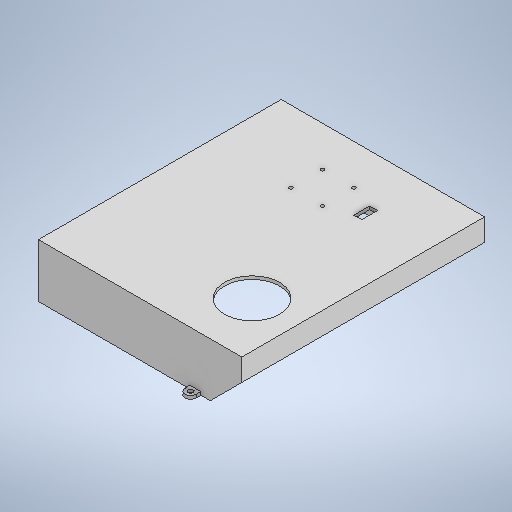
# Autodesk Inventor part: Część3
Saved by Autodesk Inventor 2025.2 (Build 292293000, 293)
## iProperties
Created: 2026-03-22
Part Number: Część3
Material: Ogólny
Document SubType Name: Modeling
Designer: janla
Density: 1 g/cm^3
Appearance: Domyślna
Author: janla
Autodesk Inventor part; units mm, degrees
ref_plane "YZ Plane" through (0, 0, 0) normal (1, 0, 0) x (0, 1, 0)
ref_plane "XZ Plane" through (0, 0, 0) normal (0, 1, 0) x (-1, 0, 0)
ref_plane "XY Plane" through (0, 0, 0) normal (0, 0, 1) x (1, 0, 0)
sketch "Szkic1" plane through (0, 0, 0) normal (0, 1, 0) x (-1, 0, 0)
  line L0 (-55.4115, -11.4249) -> (69.5885, -11.4249)
  line L1 (69.5885, -11.4249) -> (69.5885, -161.4249)
  line L2 (69.5885, -161.4249) -> (-55.4115, -161.4249)
  line L3 (-55.4115, -161.4249) -> (-55.4115, -11.4249)
  line L4 (-57.4115, -9.4249) -> (71.5885, -9.4249)
  line L5 (71.5885, -9.4249) -> (71.5885, -163.4249)
  line L6 (71.5885, -163.4249) -> (-57.4115, -163.4249)
  line L7 (-57.4115, -163.4249) -> (-57.4115, -9.4249)
  line L8 (-55.4115, -86.4249) -> (-60.9115, -86.4249)
  circle A0 centre (-60.9115, -86.4249) radius 1.65
  circle A1 centre (-60.9115, -86.4249) radius 3.5
  line L9 (-60.9115, -82.9249) -> (-57.4115, -82.9249)
  line L10 (-60.9115, -89.9249) -> (-57.4115, -89.9249)
  line L11 (-60.9115, -86.4249) -> (-27.9115, -86.4249)
  line L12 (-27.9115, -86.4249) -> (-27.9115, -166.4249)
  line L13 (-27.9115, -166.4249) -> (-27.9115, -6.4249)
  circle A2 centre (-27.9115, -6.4249) radius 1.65
  circle A3 centre (-27.9115, -166.4249) radius 1.65
  circle A4 centre (-27.9115, -6.4249) radius 3.5
  circle A5 centre (-27.9115, -166.4249) radius 3.5
  line L14 (-24.4115, -166.4249) -> (-24.4115, -163.4249)
  line L15 (-31.4115, -166.4249) -> (-31.4115, -163.4249)
  line L16 (-24.4115, -6.4249) -> (-24.4115, -9.4249)
  line L17 (-31.4115, -6.4249) -> (-31.4115, -9.4249)
  line L18 (7.0885, -9.4249) -> (7.0885, -161.4249)
  line L19 (69.5885, -11.4249) -> (42.5885, -11.4249)
  point P0 (0, 0)
  dimension "d0" = 125
  dimension "d1" = 150
  dimension "d2" = 2
  dimension "d3" = 2
  dimension "d4" = 2
  dimension "d5" = 2
  dimension "d6" = 5.5
  dimension "d7" = 3.3
  dimension "d8" = 33
  dimension "d9" = 80
  dimension "d10" = 160
  dimension "d11" = 3.3
  dimension "d12" = 3.3
  dimension "d13" = 7
  dimension "d14" = 7
  dimension "d33" = 27
  constraints: 40 end point, 12 point on line, 7 perpendicular, 6 centre point, 6 coincident, 6 point on circle, 4 horizontal, 4 parallel, 3 midpoint, 1 tangent
  measures "d0" distance between parallel lines of L1 L3
  measures "d1" distance between parallel lines of L0 L2
  measures "d2" distance between parallel lines of L5 L1
  measures "d3" distance between parallel lines of L0 L4
  measures "d4" distance between parallel lines of L6 L2
  measures "d5" distance between parallel lines of L3 L7
  measures "d6" distance of L8.start L8.end
  measures "d7" diameter of A0
  measures "d8" distance of L11.start L11.end
  measures "d9" distance of L11.end L12.end
  measures "d10" distance of L12.end L13.end
  measures "d11" diameter of A2
  measures "d12" diameter of A3
  measures "d13" diameter of A4
  measures "d14" diameter of A5
  measures "d33" distance of L0.end L19.end
extrude "Wyciągnięcie proste1" add sketch "Szkic1" along normal blind 2 contours L0 L18 L4 L5 L6 A5 L12 L2 L1 | L0 L13 A4 L4 L18 | L0 L3 L8 L7 L4 A4 L13 | A4 L4 L13 | L13 L4 A4 | L4 A4 L16 | L12 A5 L6 L7 L8 L3 L2 | L4 A4 | L4 L17 A4 | A5 L6 L12 | L12 L6 A5 | A1 L9 L7 | A1 | L7 L10 A1 | L14 A5 L6 | L6 A5 | A5 L15 L6
sketch "Szkic2" plane through (0, 2, 0) normal (0, 1, 0) x (1, 0, 0)
  line L0 (57.4115, 9.4249) -> (57.4115, 82.9249) projected
  line L1 (24.4115, 163.4249) -> (-71.5885, 163.4249) projected
  line L2 (57.4115, 9.4249) -> (-71.5885, 9.4249)
  line L3 (-71.5885, 9.4249) -> (-71.5885, 163.4249)
  line L4 (-71.5885, 163.4249) -> (57.4115, 163.4249)
  line L5 (57.4115, 163.4249) -> (57.4115, 9.4249)
  line L6 (55.4115, 11.4249) -> (-69.5885, 11.4249) projected
  line L7 (-69.5885, 11.4249) -> (55.4115, 11.4249)
  line L8 (55.4115, 11.4249) -> (55.4115, 161.4249)
  line L9 (55.4115, 161.4249) -> (-69.5885, 161.4249)
  line L10 (-69.5885, 161.4249) -> (-69.5885, 11.4249)
  point P0 (0, 0)
  point P1 (55.4115, 11.4249)
  constraints: 16 end point, 4 parallel, 2 horizontal, 2 perpendicular
extrude "Wyciągnięcie proste2" add sketch "Szkic2" along normal blind 30
sketch "Szkic3" plane through (0, 32, 0) normal (0, 1, 0) x (1, 0, 0)
  line L0 (57.4115, 9.4249) -> (57.4115, 163.4249) projected
  line L1 (-71.5885, 163.4249) -> (-71.5885, 9.4249) projected
  line L2 (57.4115, 163.4249) -> (-71.5885, 163.4249)
  line L3 (-71.5885, 163.4249) -> (-71.5885, 9.4249)
  line L4 (-71.5885, 9.4249) -> (57.4115, 9.4249)
  line L5 (57.4115, 9.4249) -> (57.4115, 163.4249)
  point P0 (0, 0)
  point P1 (-71.5885, 163.4249)
  point P2 (57.4115, 9.4249)
  constraints: 8 end point, 2 parallel, 1 horizontal, 1 perpendicular
extrude "Wyciągnięcie proste3" add sketch "Szkic3" along normal blind 2
sketch "Szkic5" plane through (57.4115, 0, -89.9249) normal (1, 0, 0) x (0, 0, -1)
  line L0 (0, 0) -> (-7, 0) projected
  line L1 (-7, 0) -> (0, 0)
  line L2 (0, 0) -> (0, 14)
  line L3 (0, 14) -> (-7, 14)
  line L4 (-7, 14) -> (-7, 0)
  line L5 (-80.5, 0) -> (-80.5, 2) projected
  line L6 (-80.5, 2) -> (-78.5, 2)
  line L7 (-78.5, 0) -> (-78.5, 32) projected
  line L8 (-7, 14) -> (-78.5, 14)
  line L9 (-78.5, 14) -> (-78.5, 2)
  line L10 (-78.5, 2) -> (-7, 2)
  line L11 (-7, 2) -> (-7, 14)
  line L12 (73.5, 0) -> (73.5, 34) projected
  line L13 (73.5, 2) -> (71.5, 2)
  line L14 (71.5, 0) -> (71.5, 32) projected
  line L15 (0, 14) -> (71.5, 14)
  line L16 (71.5, 14) -> (71.5, 2)
  line L17 (71.5, 2) -> (0, 2)
  line L18 (0, 2) -> (0, 14)
  line L19 (-7, 2) -> (-78.5, 2)
  line L20 (-78.5, 2) -> (-78.5, 0)
  line L21 (-78.5, 0) -> (-7, 0)
  line L22 (-7, 0) -> (-7, 2)
  line L23 (0, 2) -> (71.5, 2)
  line L24 (71.5, 2) -> (71.5, 0)
  line L25 (71.5, 0) -> (0, 0)
  line L26 (0, 0) -> (0, 2)
  point P0 (-89.9249, 0)
  point P1 (71.5, 14)
  point P2 (-78.5, 14)
  dimension "d24" = 14
  constraints: 44 end point, 10 parallel, 7 horizontal, 5 perpendicular, 3 point on line
  measures "d24" distance between parallel lines of L0 L3
extrude "Wyciągnięcie proste5" cut sketch "Szkic5" along normal mid plane 20
chamfer "Faza1" distance 20 angle 45 1 edges at (57.4115, 0, -10.4249)
sketch "Szkic6" plane through (-71.5885, 0, -163.4249) normal (-1, 0, 0) x (0, 0, 1)
  line L0 (0, 0) -> (154, 0) projected
  line L1 (154, 34) -> (0, 34) projected
  line L2 (0, 0) -> (154, 34)
  line L3 (0, 0) -> (0, 34) projected
  line L4 (154, 34) -> (0, 34)
  line L5 (0, 34) -> (154, 0)
  line L6 (77, 17) -> (77, 18)
  line L7 (152, 18) -> (2, 18) projected
  line L8 (77, 17) -> (77, 16)
  line L9 (77, 16) -> (80, 16)
  line L10 (80, 16) -> (74, 16)
  line L11 (74, 16) -> (80, 16)
  line L12 (80, 16) -> (80, 18)
  line L13 (80, 18) -> (74, 18)
  line L14 (74, 18) -> (74, 16)
  point P0 (163.4249, 0)
  point P1 (80, 16)
  dimension "d34" = 1
  dimension "d35" = 3
  dimension "d36" = 6
  constraints: 22 end point, 3 perpendicular, 3 point on line, 2 midpoint, 2 parallel, 1 horizontal
  measures "d34" distance of L6.start L8.end
  measures "d35" distance of L8.end L9.end
  measures "d36" distance of L9.end L10.end
extrude "Wyciągnięcie proste6" add sketch "Szkic6" along normal blind 7 contours L14 L5 L2 | L2 L8 L10 L14 | L12 L9 L8 L5 | L5 L2 L12 | L6 L7 L12 L2 | L5 L14 L7 L6
sketch "Szkic7" plane through (-71.5885, 16, -89.4249) normal (0, -1, 0) x (1, 0, 0)
  line L0 (-7, 0) -> (-7, 6) projected
  line L1 (0, 6) -> (0, 0) projected
  line L2 (-7, 0) -> (0, 6)
  line L3 (0, 6) -> (-7, 6)
  line L4 (-7, 6) -> (0, 0)
  circle A0 centre (-3.5, 3) radius 2
  point P0 (71.5885, 89.4249)
  dimension "d39" = 4
  constraints: 6 end point, 1 centre point, 1 horizontal, 1 midpoint
  measures "d39" diameter of A0
extrude "Wyciągnięcie proste7" cut sketch "Szkic7" against normal blind 7 contours A0 L4 L2 | L2 L4 A0 | A0 L2 L4 | L2 A0 L4
fillet "Zaokrąglenie powierzchni3" radius 5 1 edges at (-71.5885, 17, -89.4249)
fillet "Zaokrąglenie powierzchni4" radius 5 1 edges at (-71.5885, 17, -83.4249)
fillet "Zaokrąglenie2" radius 2 2 edges at (-78.5885, 17, -89.4249) (-78.5885, 17, -83.4249)
sketch "Szkic8" plane through (0, 34, 0) normal (0, 1, 0) x (1, 0, 0)
  line L0 (-71.5885, 94.4249) -> (-71.5885, 78.4249) projected
  line L1 (-71.5885, 78.4249) -> (55.4115, 78.4249)
  line L2 (55.4115, 161.4249) -> (55.4115, 11.4249) projected
  line L3 (0, 78.4249) -> (0, 11.4249)
  line L4 (-71.5885, 9.4249) -> (57.4115, 9.4249) projected
  line L5 (0, 44.9249) -> (57.4115, 44.9249)
  line L6 (57.4115, 9.4249) -> (57.4115, 163.4249) projected
  line L7 (57.4115, 44.9249) -> (-42.5885, 44.9249)
  circle A0 centre (-42.5885, 44.9249) radius 17.5
  line L8 (-71.5885, 86.4249) -> (55.4115, 86.4249)
  line L9 (-42.5885, 44.9249) -> (-42.5885, 9.4249)
  line L10 (24.4115, 163.4249) -> (-71.5885, 163.4249) projected
  line L11 (-42.5885, 163.4249) -> (-42.5885, 127.9249)
  line L12 (-42.5885, 127.9249) -> (0, 127.9249)
  line L13 (0, 127.9249) -> (0, 137.9249)
  line L14 (0, 137.9249) -> (-20, 137.9249)
  line L15 (-20, 137.9249) -> (-20, 117.9249)
  line L16 (-20, 117.9249) -> (0, 117.9249)
  line L17 (0, 117.9249) -> (0, 127.9249)
  circle A1 centre (-20, 117.9249) radius 1.1
  circle A2 centre (-20, 137.9249) radius 1.1
  circle A3 centre (0, 137.9249) radius 1.1
  circle A4 centre (0, 117.9249) radius 1.1
  line L18 (-71.5885, 163.4249) -> (-71.5885, 9.4249) projected
  line L19 (-71.5885, 44.9249) -> (28.4115, 44.9249)
  circle A5 centre (28.4115, 44.9249) radius 17.5
  point P0 (0, 0)
  dimension "d45" = 100
  dimension "d46" = 35
  dimension "d47" = 35.5
  dimension "d48" = 10
  dimension "d49" = 20
  dimension "d50" = 20
  dimension "d51" = 2.2
  dimension "d52" = 2.2
  dimension "d53" = 2.2
  dimension "d54" = 2.2
  dimension "d57" = 100
  dimension "d58" = 35
  constraints: 28 end point, 11 point on line, 7 perpendicular, 6 centre point, 6 coincident, 3 midpoint, 2 horizontal, 1 parallel
  measures "d45" distance of L5.end L7.end
  measures "d46" diameter of A0
  measures "d47" distance of L11.start L11.end
  measures "d48" distance of L12.end L13.end
  measures "d49" distance of L13.end L14.end
  measures "d50" distance of L14.end L15.end
  measures "d51" diameter of A1
  measures "d52" diameter of A2
  measures "d53" diameter of A3
  measures "d54" diameter of A4
  measures "d57" distance of L19.start L19.end
  measures "d58" diameter of A5
extrude "Wyciągnięcie proste8" cut sketch "Szkic8" against normal blind 7 contours A5 L5 | L5 A5 | A2 L14 L15 | L15 L14 A2 | A1 L16 L15 | L15 L16 A1 | A3 L14 L13 | L13 L14 A3 | A4 L16 L17 | L17 L16 A4
sketch "Szkic9" plane through (0, 34, 0) normal (0, 1, 0) x (1, 0, 0)
  circle A0 centre (0, 137.9249) radius 1.1 projected
  circle A1 centre (0, 117.9249) radius 1.1 projected
  line L0 (0, 137.9249) -> (0, 117.9249)
  line L1 (0, 117.9249) -> (0, 127.9249)
  line L2 (0, 127.9249) -> (20, 127.9249)
  line L3 (20, 127.9249) -> (20, 132.9249)
  line L4 (20, 132.9249) -> (20, 122.9249)
  line L5 (20, 122.9249) -> (15, 122.9249)
  line L6 (15, 122.9249) -> (15, 132.9249)
  line L7 (15, 132.9249) -> (20, 132.9249)
  point P0 (0, 0)
  dimension "d59" = 20
  dimension "d60" = 5
  dimension "d61" = 5
  constraints: 16 end point, 4 perpendicular, 2 vertical, 1 midpoint, 1 point on line
  measures "d59" distance of L1.end L2.end
  measures "d60" distance of L2.end L3.end
  measures "d61" distance of L4.end L5.end
extrude "Wyciągnięcie proste9" cut sketch "Szkic9" against normal blind 7 contours L6 L7 L3 L2 | L2 L4 L5 L6
